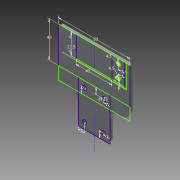
# Autodesk Inventor part: OuterBar
Saved by Autodesk Inventor 2014 SP1 (Build 180222100, 222)
## iProperties
Created: 2014-06-07
Part Number: OuterBar
Material: Generic
Document SubType Name: Modeling
Designer: Erin
Density: 1 g/cm^3
Appearance: Default
Author: Erin
Autodesk Inventor part; units mm, degrees
note: some values were not read from the file. Chosen so that the rebuilt part matches the saved one: sketch regions of "Extrusion8".
ref_plane "YZ Plane" through (0, 0, 0) normal (1, 0, 0) x (0, 1, 0)
ref_plane "XY Plane" through (0, 0, 0) normal (0, 0, 1) x (1, 0, 0)
sketch "Sketch1" plane through (0, 0, 0) normal (0, 1, 0) x (-1, 0, 0)
  line L0 (-51.65, 23.5) -> (51.65, 23.5)
  line L1 (54.65, 20.5) -> (54.65, -20.5)
  line L2 (51.65, -23.5) -> (-51.65, -23.5)
  line L3 (-54.65, -20.5) -> (-54.65, 20.5)
  circle A0 centre (-47.65, 16.5) radius 2.25
  circle A1 centre (47.65, 16.5) radius 2.25
  circle A2 centre (-47.65, 16.5) radius 26.75 construction
  circle A3 centre (-10.7, 16.5) radius 2.25
  circle A4 centre (-10.7, 16.5) radius 11.2 construction
  line L4 (-21.9, 16.5) -> (-21.9, 6.8604)
  line L5 (-20.9, 16.5) -> (-20.9, 6.8604)
  circle A5 centre (10.7, 16.5) radius 2.25
  circle A6 centre (10.7, 16.5) radius 11.2 construction
  line L6 (-0.5, 16.5) -> (-0.5, 5.694)
  line L7 (0.5, 16.5) -> (0.5, 5.694)
  circle A7 centre (47.65, 16.5) radius 26.75 construction
  line L8 (20.9, 16.5) -> (20.9, 5.8426)
  line L9 (21.9, 16.5) -> (21.9, 5.8426)
  arc A8 (-51.65, 23.5) -> (-54.65, 20.5) centre (-51.65, 20.5) ccw
  arc A9 (-54.65, -20.5) -> (-51.65, -23.5) centre (-51.65, -20.5) ccw
  arc A10 (54.65, 20.5) -> (51.65, 23.5) centre (51.65, 20.5) ccw
  arc A11 (51.65, -23.5) -> (54.65, -20.5) centre (51.65, -20.5) ccw
  line L10 (-84.9483, 16.5) -> (77.5332, 16.5) construction
  line L11 (-54.65, 0) -> (54.65, 0)
  line L12 (10.7, 30.5) -> (10.7, -33.5) construction
  circle A12 centre (10.7, -16.5) radius 2.25
  line L13 (5, -8.5) -> (18, -8.5) construction
  line L14 (3.7, -4.5) -> (3.7, -33.5) construction
  line L15 (-6.3, -4.5) -> (-6.3, -33.5) construction
  line L16 (-1.3, -33.5) -> (-1.3, -4.5) construction
  circle A13 centre (-1.3, -38.9) radius 2.25
  circle A14 centre (-1.3, -8.5) radius 2.25
  line L17 (-17.7373, -23.5) -> (14.2274, -23.5)
  line L18 (14.2274, -23.5) -> (14.2274, -45.3565)
  line L19 (14.2274, -45.3565) -> (-17.7373, -45.3565)
  line L20 (-17.7373, -45.3565) -> (-17.7373, -23.5)
  line L21 (-40.65, 5) -> (-30.65, 5)
  line L22 (-30.65, 5) -> (-30.65, -5)
  line L23 (-30.65, -5) -> (-40.65, -5)
  line L24 (-40.65, -5) -> (-40.65, 5)
  line L25 (-42.65, -7) -> (-28.65, -7)
  line L26 (-28.65, -7) -> (-28.65, 7)
  line L27 (-28.65, 7) -> (-42.65, 7)
  line L28 (-42.65, 7) -> (-42.65, -7)
  point P0 (0, 0)
  point P1 (-54.65, 23.5)
  point P2 (-54.65, -23.5)
  point P3 (0, 23.5)
  point P4 (-35.65, 5)
  point P5 (-30.65, 0)
  dimension "d5" = 53.5
  dimension "d12" = 53.5
  dimension "d1" = 4.5
  dimension "d2" = 7
  dimension "d3" = 4.5
  dimension "d4" = 7
  dimension "d6" = 4.5
  dimension "d7" = 22.4
  dimension "d8" = 1
  dimension "d9" = 4.5
  dimension "d10" = 22.4
  dimension "d11" = 1
  dimension "d13" = 1
  dimension "d14" = 3
  dimension "d23" = 16.5
  dimension "d24" = 7
  dimension "d27" = 8
  dimension "d28" = 7
  dimension "d29" = 10
  dimension "d30" = 5
  dimension "d31" = 4.5
  dimension "d32" = 4.5
  dimension "d33" = 30.4
  dimension "d38" = 0
  dimension "d40" = 10
  dimension "d41" = 10
  dimension "d43" = 2
  dimension "d47" = 12
  constraints: 58 end point, 17 parallel, 13 centre point, 12 point on circle, 12 point on line, 12 tangent, 8 perpendicular, 5 midpoint, 4 coincident, 4 horizontal alignment, 3 equal radius, 3 horizontal, 2 vertical, 1 symmetric about line, 1 vertical alignment, 8 other
  measures "d1" diameter of A0
  measures "d2" distance from line of A0.centre L3
  measures "d3" diameter of A1
  measures "d4" distance from line of A1.centre L1
  measures "d6" diameter of A3
  measures "d7" diameter of A4
  measures "d8" distance between parallel lines of L5 L4
  measures "d9" diameter of A5
  measures "d10" diameter of A6
  measures "d11" distance between parallel lines of L7 L6
  measures "d13" distance between parallel lines of L9 L8
  measures "d14" radius of A8
  measures "d23" distance between parallel lines of L11 L10
  measures "d24" distance between parallel lines of L10 L0
  measures "d27" distance from line of A12.centre L13
  measures "d28" distance between parallel lines of L14 L12
  measures "d29" distance between parallel lines of L15 L14
  measures "d30" distance between parallel lines of L14 L16
  measures "d31" diameter of A13
  measures "d32" diameter of A14
  measures "d33" distance of A13.centre A14.centre
  measures "d38" distance from line of A14.centre L13
  measures "d40" distance of L23.end L21.start
  measures "d41" distance of L21.start L21.end
  measures "d43" distance between parallel lines of L25 L23
  measures "d47" horizontal distance of point (-35.65, 5) A0.centre
ref_plane "Work Plane1" through (0, 3, 0) normal (0, 1, 0) x (-1, 0, 0)
sketch "Sketch3" plane through (0, 3, 0) normal (0, 1, 0) x (-1, 0, 0)
  circle A0 centre (-10.7, -16.5) radius 2.25
  circle A1 centre (10.7, -16.5) radius 2.25
  circle A2 centre (10.7, 16.5) radius 2.25
  circle A3 centre (-10.7, 16.5) radius 2.25
  line L0 (-17.7, -23.5) -> (17.7, -23.5)
  line L1 (17.7, 23.5) -> (-17.7, 23.5)
  line L2 (-17.7, 23.5) -> (-17.7, -23.5)
  line L3 (17.7, 23.5) -> (17.7, -23.5)
  line L4 (-40, 23.5) -> (40, 23.5)
  line L5 (40, 23.5) -> (40, 63.5)
  line L6 (40, 63.5) -> (-40, 63.5)
  line L7 (-40, 63.5) -> (-40, 23.5)
  line L8 (-20, 63.5) -> (20, 63.5)
  line L9 (20, 63.5) -> (20, 40)
  line L10 (20, 40) -> (-20, 40)
  line L11 (-20, 40) -> (-20, 63.5)
  line L12 (0, 0) -> (0, -39.7707) construction
  line L13 (0, 40) -> (0, 63.5) construction
  line L14 (-40, 23.5) -> (-40, 9.5)
  line L15 (-40, 9.5) -> (40, 9.5)
  line L16 (40, 9.5) -> (40, 23.5)
  circle A4 centre (-27, 58.5) radius 2.25
  line L17 (-20, 40) -> (-34, 40)
  line L18 (-34, 40) -> (-34, 63.5)
  line L19 (-34, 63.5) -> (-20, 63.5)
  line L20 (-20, 63.5) -> (-20, 40)
  circle A5 centre (-27, 45) radius 2.25
  line L21 (-20, 38) -> (-34, 38)
  line L22 (-36, 38) -> (-36, 63.5)
  line L23 (-20, 38) -> (-20, 40)
  line L24 (-36, 63.5) -> (-34, 63.5)
  line L25 (20, 40) -> (20, 38)
  line L26 (-34, 38) -> (-36, 38)
  line L27 (-20, 38) -> (20, 38)
  line L28 (-36, 54.8338) -> (-34, 54.8338)
  point P0 (0, 63.5)
  point P1 (0, 23.5)
  point P2 (-27, 63.5)
  dimension "d67" = 7
  dimension "d73" = 7
  dimension "d74" = 7
  dimension "d84" = 7
  dimension "d86" = 7
  dimension "d87" = 40
  dimension "d88" = 80
  dimension "d91" = 40
  dimension "d92" = 23.5
  dimension "d96" = 4.5
  dimension "d97" = 7
  dimension "d98" = 4.5
  dimension "d99" = 7
  dimension "d100" = 5
  dimension "d101" = 4.5
  dimension "d102" = 7
  dimension "d103" = 5
  dimension "d104" = 2
  constraints: 58 end point, 11 perpendicular, 8 parallel, 6 centre point, 5 midpoint, 5 point on line, 3 horizontal, 2 collinear, 2 vertical alignment, 1 vertical, 4 other
  measures "d67" distance from line of A3.centre L1
  measures "d73" distance from line of A0.centre L2
  measures "d74" distance from line of A1.centre L3
  measures "d84" distance from line of A0.centre L0
  measures "d86" distance from line of A3.centre L2
  measures "d87" distance of L4.end L5.end
  measures "d88" distance of L5.end L6.end
  measures "d91" distance of L9.end L10.end
  measures "d92" distance of L8.end L9.end
  measures "d96" diameter of A3
  measures "d97" distance from line of A2.centre L15
  measures "d98" diameter of A4
  measures "d99" distance from line of A4.centre L18
  measures "d100" distance from line of L19 A4.centre
  measures "d101" diameter of A5
  measures "d102" distance from line of A5.centre L18
  measures "d103" distance from line of A5.centre L17
  measures "d104" distance between parallel lines of L21 L17
extrude "Extrusion8" add sketch "Sketch3" along normal blind 3 contours L2 L15 L3 L0 | L15 L14 L4 L2 | L2 L1 L3 L15 | L3 L4 L16 L15 | L4 L7 L6 L22 L26 L21 L27 L25 L9 L5 L1 | L6 L18 L28 L22 | L9 L10 L11 L6 | L6 L11 L17 L18 | L28 L18 L17 L23 L21 L26 L22 | L25 L27 L23 L10 | A4 | A5
extrude "Extrusion9" cut sketch "Sketch3" along normal blind 1 contours L28 L18 L17 L23 L21 L26 L22 | L25 L27 L23 L10
extrude "Extrusion10" cut sketch "Sketch3" along normal blind 10 contours A4 | A5
mirror "Mirror4" about plane through (0, 0, 0) normal (1, 0, 0) of "Extrusion9", "Extrusion10"
fillet "Fillet3" radius 10 4 edges at (-40, 4.5, 9.5) (-17.7, 4.5, 9.5) (17.7, 4.5, 9.5) (40, 4.5, 9.5)
fillet "Fillet4" radius 4 4 edges at (-40, 4.5, 63.5) (40, 4.5, 63.5) (-17.7, 4.5, -23.5) (17.7, 4.5, -23.5)
body "Solid2"
